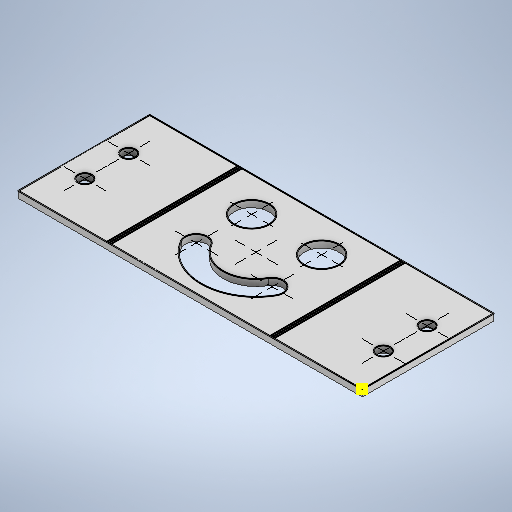
# Autodesk Inventor part: Head2
Saved by Autodesk Inventor 2026.1 (Build 301233000, 233)
## iProperties
Created: 2025-08-16
Part Number: Head2
Material: Generic
Document SubType Name: Modeling
Designer: chris
Density: 1 g/cm^3
Appearance: Default
Author: chris
Autodesk Inventor part; units mm, degrees
ref_plane "YZ Plane" through (0, 0, 0) normal (1, 0, 0) x (0, 1, 0)
ref_plane "XZ Plane" through (0, 0, 0) normal (0, 1, 0) x (-1, 0, 0)
ref_plane "XY Plane" through (0, 0, 0) normal (0, 0, 1) x (1, 0, 0)
sketch "Sketch1" plane through (0, 0, 0) normal (0, 1, 0) x (-1, 0, 0)
  line L0 (20.6396, 0) -> (20.6396, -30)
  line L1 (57.9189, -30) -> (57.9189, 0)
  arc A0 (50.1046, -8.75) -> (28.454, -8.75) centre (39.2793, -15) ccw
  arc A1 (28.454, -8.75) -> (32.7841, -11.25) centre (30.619, -10) ccw
  arc A2 (45.7745, -11.25) -> (32.7841, -11.25) centre (39.2793, -15) ccw
  arc A3 (45.7745, -11.25) -> (50.1046, -8.75) centre (47.9395, -10) ccw
  circle A4 centre (47.2793, -22) radius 4
  circle A5 centre (31.2793, -22) radius 4
  circle A6 centre (73.3686, -10) radius 1.55
  circle A7 centre (5.19, -10) radius 1.55
  circle A8 centre (73.3686, -20) radius 1.55
  circle A9 centre (5.19, -20) radius 1.55
  line L2 (0, -30) -> (0, 0)
  line L3 (78.5586, -30) -> (0, -30)
  line L4 (0, 0) -> (78.5586, 0)
  line L5 (78.5586, 0) -> (78.5586, -30)
  line L6 (58.3686, 0) -> (58.3686, -30)
  line L7 (57.4693, -30) -> (57.4693, 0)
  line L8 (21.0893, 0) -> (21.0893, -30)
  line L9 (20.19, -30) -> (20.19, 0)
  constraints: 20 end point, 12 point on line, 10 centre point, 8 point on circle, 8 vertical, 7 parallel, 5 equal radius, 3 tangent, 2 horizontal, 2 perpendicular, 40 other
extrude "Extrusion1" add sketch "Sketch1" against normal blind 1.5
body "Solid1"
